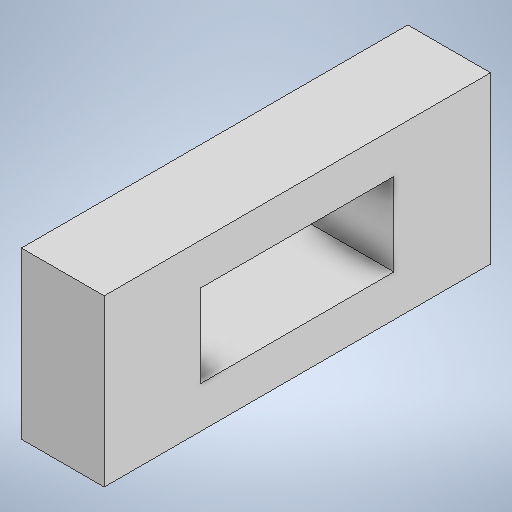
# Autodesk Inventor part: encaixe do suporte do motor
Saved by Autodesk Inventor 2025.2 (Build 292293000, 293)
## iProperties
Created: 2025-05-20
Part Number: encaixe do suporte do motor
Material: Genérico
Document SubType Name: Modeling
Designer: erick
Density: 1 g/cm^3
Appearance: Padrão
Author: erick
Autodesk Inventor part; units mm, degrees
ref_plane "YZ Plane" through (0, 0, 0) normal (1, 0, 0) x (0, 1, 0)
ref_plane "XZ Plane" through (0, 0, 0) normal (0, 1, 0) x (-1, 0, 0)
ref_plane "XY Plane" through (0, 0, 0) normal (0, 0, 1) x (1, 0, 0)
sketch "Esboço1" plane through (0, 0, 0) normal (1, 0, 0) x (0, 1, 0)
  line L0 (-6, 14) -> (6, 14)
  line L1 (6, 14) -> (6, -14)
  line L2 (6, -14) -> (-6, -14)
  line L3 (-6, -14) -> (-6, 14)
  line L4 (-6, 14) -> (6, -14) construction
  line L5 (6, 14) -> (-6, -14) construction
  point P0 (0, 0)
  dimension "d0" = 28
  dimension "d1" = 12
  constraints: 12 end point, 2 midpoint, 2 parallel, 1 horizontal, 1 perpendicular
  measures "d0" distance of L0.end L1.end
  measures "d1" distance of L1.end L2.end
extrude "Extrusão1" add sketch "Esboço1" along normal mid plane 6
sketch "Esboço2" plane through (3, 0, 0) normal (1, 0, 0) x (0, 0, -1)
  line L0 (-7, -3) -> (7, -3)
  line L1 (7, -3) -> (7, 3)
  line L2 (7, 3) -> (-7, 3)
  line L3 (-7, 3) -> (-7, -3)
  line L4 (-7, -3) -> (7, 3) construction
  line L5 (7, -3) -> (-7, 3) construction
  point P0 (0, 0)
  dimension "d4" = 14
  dimension "d5" = 6
  constraints: 12 end point, 2 midpoint, 2 parallel, 1 horizontal, 1 perpendicular
  measures "d4" distance of L1.end L2.end
  measures "d5" distance of L0.end L1.end
extrude "Extrusão2" cut sketch "Esboço2" against normal through all
